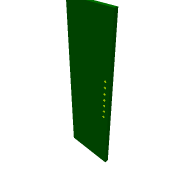
# Autodesk Inventor part: pcb
Saved by Autodesk Inventor 2016 (Build 200138000, 138)
## iProperties
Created: 2015-07-07
Part Number: pcb
Material: Generic
Document SubType Name: Modeling
Designer: Sebastian
Density: 1 g/cm^3
Appearance: Default
Mass: 2 g
Surface Area: 27.6619 cm^2
Volume: 2 cm^3
GlobalPropertyList: <PropertyList/>
Author: Sebastian
Autodesk Inventor part; units mm, degrees
ref_plane "YZ Plane" through (0, 0, 0) normal (1, 0, 0) x (0, 1, 0)
ref_plane "XZ Plane" through (0, 0, 0) normal (0, 1, 0) x (-1, 0, 0)
ref_plane "XY Plane" through (0, 0, 0) normal (0, 0, 1) x (1, 0, 0)
sketch "Sketch1" plane through (0, 0, 0) normal (0, 1, 0) x (-1, 0, 0)
  line L0 (0, 0) -> (19.685, 0)
  line L1 (19.685, 0) -> (19.685, -63.5)
  line L2 (19.685, -63.5) -> (0, -63.5)
  line L3 (0, -63.5) -> (0, 0)
  circle A0 centre (2, -24.13) radius 0.5
  circle A1 centre (2, -26.67) radius 0.5
  circle A2 centre (2, -29.21) radius 0.5
  circle A3 centre (2, -31.75) radius 0.5
  circle A4 centre (2, -34.29) radius 0.5
  circle A5 centre (2, -36.83) radius 0.5
  circle A6 centre (2, -39.37) radius 0.5
  dimension "d0" = 19.685
  dimension "d1" = 63.5
  dimension "d4" = 1
  dimension "d5" = 1
  dimension "d6" = 1
  dimension "d7" = 1
  dimension "d8" = 1
  dimension "d9" = 1
  dimension "d10" = 2.54
  dimension "d11" = 2.54
  dimension "d12" = 2.54
  dimension "d13" = 2.54
  dimension "d14" = 2.54
  dimension "d19" = 2
  dimension "d20" = 1
  dimension "d21" = 2.54
  dimension "d22" = 31.75
  constraints: 8 end point, 7 centre point, 2 parallel, 1 horizontal, 1 perpendicular
  measures "d0" distance of L1.end L2.end
  measures "d1" distance of L0.end L1.end
  measures "d4" diameter of A0
  measures "d5" diameter of A1
  measures "d6" diameter of A2
  measures "d7" diameter of A3
  measures "d8" diameter of A4
  measures "d9" diameter of A5
  measures "d10" distance of A1.centre A0.centre
  measures "d11" distance of A2.centre A1.centre
  measures "d12" distance of A3.centre A2.centre
  measures "d13" distance of A4.centre A3.centre
  measures "d14" distance of A4.centre A5.centre
  measures "d19" distance from line of L3 A3.centre
  measures "d20" diameter of A6
  measures "d21" distance of A5.centre A6.centre
  measures "d22" distance from line of L0 A3.centre
extrude "Extrusion3" add sketch "Sketch1" along normal blind 1.6
sketch "Sketch2" plane through (0, 0, 0) normal (0, -1, 0) x (1, 0, 0)
  circle A0 centre (-2, -24.13) radius 0.5 projected
sketch "Sketch3" plane through (0, 0, 0) normal (0, -1, 0) x (1, 0, 0)
  circle A0 centre (-2, -26.67) radius 0.5 projected
sketch "Sketch4" plane through (0, 0, 0) normal (0, -1, 0) x (1, 0, 0)
  circle A0 centre (-2, -29.21) radius 0.5 projected
sketch "Sketch5" plane through (0, 0, 0) normal (0, -1, 0) x (1, 0, 0)
  circle A0 centre (-2, -31.75) radius 0.5 projected
sketch "Sketch6" plane through (0, 0, 0) normal (0, -1, 0) x (1, 0, 0)
  circle A0 centre (-2, -34.29) radius 0.5 projected
sketch "Sketch7" plane through (0, 0, 0) normal (0, -1, 0) x (1, 0, 0)
  circle A0 centre (-2, -36.83) radius 0.5 projected
sketch "Sketch8" plane through (0, 0, 0) normal (0, -1, 0) x (1, 0, 0)
  circle A0 centre (-2, -39.37) radius 0.5 projected
body "Solid3"
